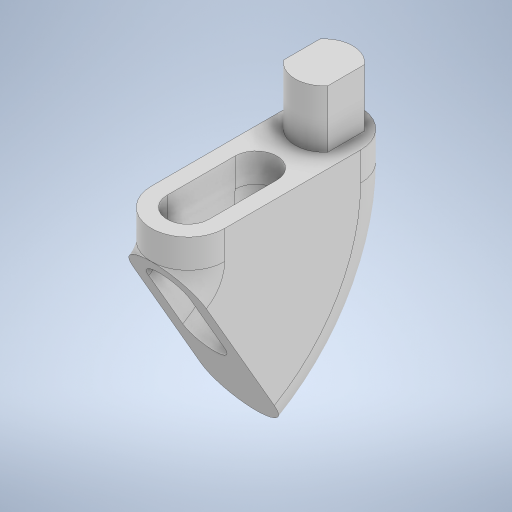
# Autodesk Inventor part: esercizio2 02-27-2023
Saved by Autodesk Inventor 2023 (Build 270158000, 158)
## iProperties
Created: 2023-02-27
Part Number: esercizio2 02-27-2023
Material: Generico
Document SubType Name: Modeling
Designer: Admin
Density: 1 g/cm^3
Appearance: Default
Author: Admin
Autodesk Inventor part; units mm, degrees
ref_plane "YZ Plane" through (0, 0, 0) normal (1, 0, 0) x (0, 1, 0)
ref_plane "XZ Plane" through (0, 0, 0) normal (0, 1, 0) x (-1, 0, 0)
ref_plane "XY Plane" through (0, 0, 0) normal (0, 0, 1) x (1, 0, 0)
sketch "Schizzo1" plane through (0, 0, 0) normal (0, 1, 0) x (-1, 0, 0)
  line L0 (0, 0) -> (0, -52)
  arc A0 (0, -52) -> (28, -52) centre (14, -52) ccw
  line L1 (28, -52) -> (28, 0)
  arc A1 (28, 0) -> (0, 0) centre (14, 0) ccw
  line L2 (22, 0) -> (22, -26)
  arc A2 (22, 0) -> (6, 0) centre (14, 0) ccw
  line L3 (6, 0) -> (6, -26)
  arc A3 (6, -26) -> (22, -26) centre (14, -26) ccw
  circle A4 centre (14, -52) radius 11
  line L4 (22.5, -45.0179) -> (22.5, -58.9821)
  line L5 (5.5, -45.0179) -> (5.5, -58.9821)
  dimension "d0" = 22
  dimension "d3" = 8.5
  dimension "d4" = 8.5
  dimension "d5" = 28
  dimension "d6" = 16
  dimension "d7" = 26
  dimension "d8" = 52
  constraints: 12 end point, 12 point on circle, 8 tangent, 5 centre point, 4 vertical, 1 coincident, 1 concentric, 1 parallel
  measures "d0" diameter of A4
  measures "d3" distance from line of A0.centre L4
  measures "d4" distance from line of A0.centre L5
  measures "d5" distance between parallel lines of L0 L1
  measures "d6" distance between parallel lines of L3 L2
  measures "d7" distance of L3.start L3.end
  measures "d8" distance of L0.start L0.end
extrude "Estrusione1" add sketch "Schizzo1" along normal blind 33 contours L4 A4 L5
extrude "Estrusione2" add sketch "Schizzo1" along normal blind 11 contours A1 L1 A0 L0 | A4 L4 | L5 A4
sketch "Schizzo4" plane through (0, 0, 0) normal (0, -1, 0) x (1, 0, 0)
  arc A0 (0, 0) -> (-28, 0) centre (-14, 0) ccw projected
  line L0 (-28, 0) -> (-28, -51.655)
  arc A1 (-28, -52) -> (0, -52) centre (-14, -52) ccw projected
  line L1 (-28, -51.655) -> (-28, -52)
  arc A2 (-28, -52) -> (0, -52) centre (-14, -52) ccw
  line L2 (0, 0) -> (0, -52) projected
  line L3 (0, -52) -> (0, 0)
  arc A3 (0, 0) -> (-28, 0) centre (-14, 0) ccw
  line L4 (0, 14) -> (-28, 14)
  arc A4 (-22, -26) -> (-6, -26) centre (-14, -26) ccw projected
  line L5 (-22, -26) -> (-22, 0)
  arc A5 (-22, -26) -> (-6, -26) centre (-14, -26) ccw
  line L6 (-6, -26) -> (-6, 0) projected
  line L7 (-6, -26) -> (-6, 0)
  arc A6 (-6, 0) -> (-22, 0) centre (-14, 0) ccw
  constraints: 12 end point, 11 tangent, 8 point on circle, 4 centre point, 2 collinear, 2 vertical, 1 horizontal, 1 parallel
revolve "Rivoluzione1" add sketch "Schizzo4" angle 60 about axis through (0, 0, 14) along (-1, 0, 0)
